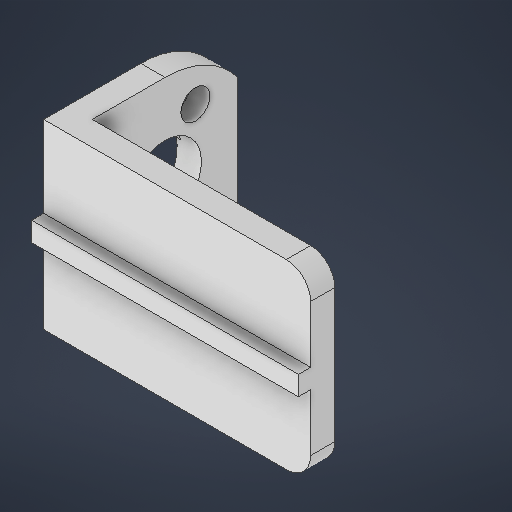
# Autodesk Inventor part: Trzymak
Saved by Autodesk Inventor 2026 (Build 300175000, 175)
## iProperties
Created: 2025-04-24
Part Number: Trzymak
Material: Generic
Document SubType Name: Modeling
Designer: isan
Density: 1 g/cm^3
Appearance: Default
Author: isan
Autodesk Inventor part; units mm, degrees
ref_plane "YZ Plane" through (0, 0, 0) normal (1, 0, 0) x (0, 1, 0)
ref_plane "XZ Plane" through (0, 0, 0) normal (0, 1, 0) x (-1, 0, 0)
ref_plane "XY Plane" through (0, 0, 0) normal (0, 0, 1) x (1, 0, 0)
sketch "Sketch1" plane through (0, 0, 0) normal (0, 1, 0) x (-1, 0, 0)
  line L0 (-11, 7.5) -> (11, 7.5)
  line L1 (11, 7.5) -> (11, -7.5)
  line L2 (11, -7.5) -> (-11, -7.5)
  line L3 (-11, -7.5) -> (-11, 7.5)
  line L4 (-11, 7.5) -> (11, -7.5) construction
  line L5 (11, 7.5) -> (-11, -7.5) construction
  point P0 (0, 0)
  dimension "d0" = 22
  dimension "d1" = 15
  constraints: 12 end point, 2 midpoint, 2 parallel, 1 horizontal, 1 perpendicular
  measures "d0" distance of L1.end L2.end
  measures "d1" distance of L0.end L1.end
extrude "Extrusion1" add sketch "Sketch1" along normal blind 2
sketch "Sketch2" plane through (0, 2, 0) normal (0, 1, 0) x (1, 0, 0)
  line L0 (-11, 7.5) -> (-11, -7.5) projected
  line L1 (-11, -7.5) -> (-9, -7.5)
  line L2 (-9, -7.5) -> (-9, 7.5)
  line L3 (-9, 7.5) -> (-11, 7.5)
  line L4 (-11, 7.5) -> (-11, -7.5)
  point P0 (0, 0)
  point P1 (-11, 0)
  dimension "d4" = 2
  dimension "d5" = 15
  constraints: 8 end point, 2 midpoint, 2 parallel, 1 horizontal, 1 perpendicular
  measures "d4" distance of L2.end L3.end
  measures "d5" distance of L1.end L2.end
extrude "Extrusion2" add sketch "Sketch2" along normal blind 12
sketch "Sketch3" plane through (-9, 2, 7.5) normal (1, 0, 0) x (0, 0, -1)
  circle A0 centre (7.5, 6) radius 3
  line L0 (0, 12) -> (15, 12) projected
  line L1 (15, 0) -> (15, 12) projected
  circle A1 centre (3.1699, 8.5) radius 1.2
  line L2 (0, -2) -> (0, 12) projected
  line L3 (0, 6) -> (15, 6) construction
  line L4 (0.8753, 9.8248) -> (14.1247, 2.1752) construction
  circle A2 centre (11.8301, 3.5) radius 1.2
  point P0 (7.5, -2)
  point P1 (7.5, 6)
  dimension "d8" = 6
  dimension "d9" = 6
  dimension "d10" = 7.5
  dimension "d11" = 2.4
  dimension "d12" = -30
  dimension "d13" = 5
  dimension "d14" = 2.4
  dimension "d15" = 5
  constraints: 4 end point, 3 centre point, 3 midpoint, 3 point on line
  measures "d8" diameter of A0
  measures "d9" distance from line of L0 A0.centre
  measures "d10" distance from line of L1 A0.centre
  measures "d11" diameter of A1
  measures "d12" angle of L3 L4
  measures "d13" distance of A0.centre A1.centre
  measures "d14" diameter of A2
  measures "d15" distance of A0.centre A2.centre
extrude "Extrusion3" cut sketch "Sketch3" against normal blind 2
sketch "Sketch4" plane through (-11, 0, -7.5) normal (-1, 0, 0) x (0, 0, 1)
  circle A0 centre (7.5, 8) radius 3 projected
  circle A1 centre (7.5, 8) radius 7.5
  line L0 (0, 0) -> (0, 14) projected
  circle A2 centre (7.5, 8) radius 12.6892
  line L1 (7.5, 8) -> (-5.1892, 8)
  line L2 (7.5, 8) -> (20.1892, 8)
  point P0 (7.5, 0)
  point P1 (15, 8)
  point P2 (0, 8)
  dimension "d18" = 15
  constraints: 4 end point, 2 centre point, 2 coincident, 2 point on circle, 1 horizontal, 1 point on line, 1 tangent
  measures "d18" diameter of A1
extrude "Extrusion4" cut sketch "Sketch4" against normal blind 2 contours A1 L1 A2 L2 picked at (-3.2639, 9.6105)
sketch "Sketch5" plane through (-11, 0, -7.5) normal (-1, 0, 0) x (0, 0, 1)
  circle A0 centre (3.1699, 5.5) radius 1.2 projected
  circle A1 centre (11.8301, 10.5) radius 1.2 projected
  line L0 (3.1699, 5.5) -> (11.8301, 10.5) construction
  line L1 (4.2199, 3.6813) -> (12.8801, 8.6813)
  line L2 (10.7801, 12.3187) -> (2.1199, 7.3187)
  arc A2 (2.1199, 7.3187) -> (4.2199, 3.6813) centre (3.1699, 5.5) ccw
  arc A3 (12.8801, 8.6813) -> (10.7801, 12.3187) centre (11.8301, 10.5) ccw
  point P0 (7.5, 0)
  point P1 (7.5, 8)
  constraints: 8 end point, 4 point on circle, 4 tangent, 2 centre point, 1 midpoint, 1 parallel
extrude "Extrusion6" cut sketch "Sketch5" against normal blind 0.4
sketch "Sketch7" plane through (0, 0, 0) normal (0, -1, 0) x (1, 0, 0)
  line L0 (-11, -7.5) -> (-11, 7.5) projected
  line L1 (-11, 0.8) -> (11, 0.8)
  line L2 (11, 0.8) -> (11, -0.8)
  line L3 (11, -0.8) -> (-11, -0.8)
  line L4 (-11, -0.8) -> (-11, 0.8)
  line L5 (11, 7.5) -> (11, -7.5) projected
  point P0 (0, 0)
  point P1 (-11, -0.8)
  dimension "d27" = 1.6
  dimension "d28" = 0.8
  constraints: 8 end point, 2 parallel, 1 collinear, 1 horizontal, 1 perpendicular, 1 point on line
  measures "d27" distance of L1.end L2.end
  measures "d28" distance from line of point (0, 0) L1
extrude "Extrusion7" add sketch "Sketch7" along normal blind 1
fillet "Fillet1" radius 2 2 edges at (11, 1, -7.5) (11, 1, 7.5)
body "Solid1"
